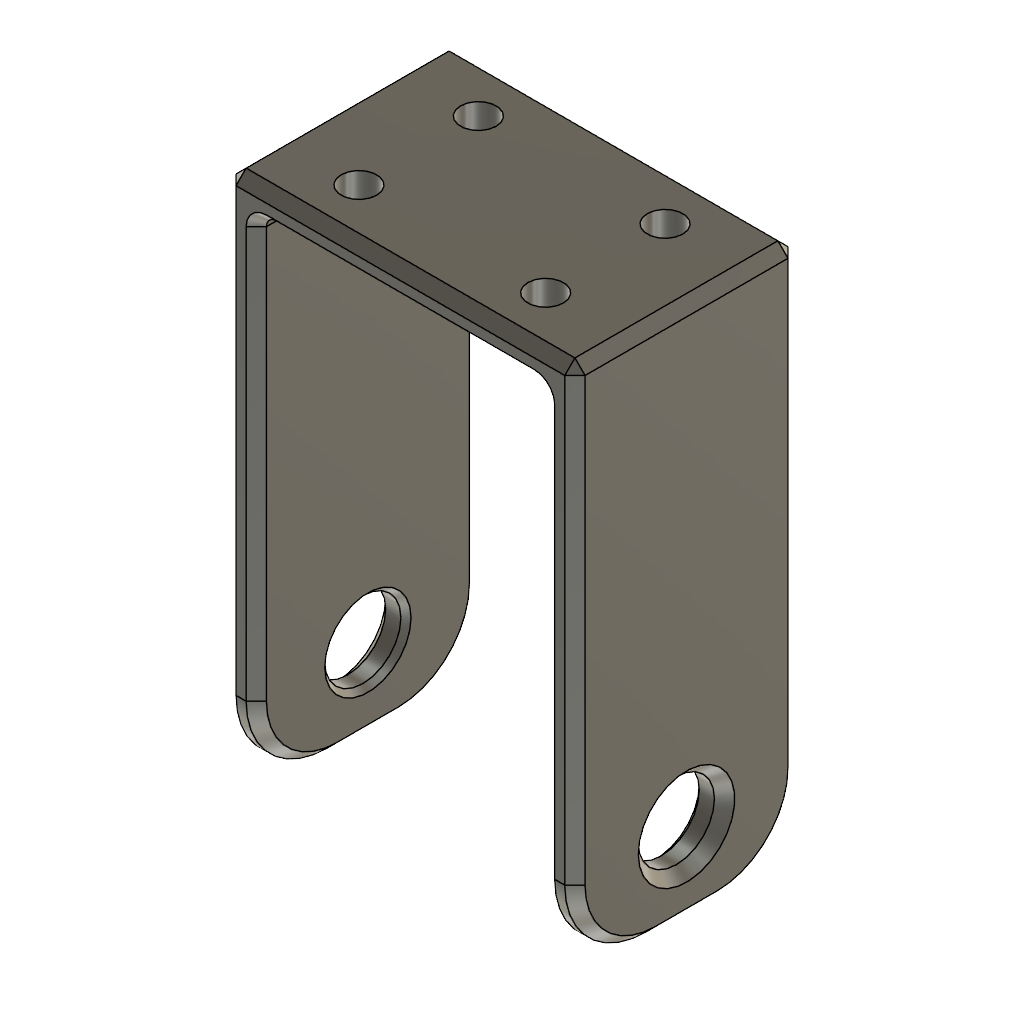
ZoMa_Bracket_omni_wheel_v001 (Autodesk Fusion 360 design; units mm, degrees)
part number: 2026-08-14-10-01-13-584
part number: 2026-08-14-10-48-38-713
part number: 2026-08-14-10-49-42-886
part number: 2026-08-14-10-49-47-612
part number: 2026-08-14-10-49-51-894
part number: 2026-08-14-11-24-35-038
part number: 2026-08-18-17-26-55-880
part number: 2026-08-18-17-40-12-881
part number: 2026-08-19-15-49-04-728
part number: 2026-08-21-16-16-46-057
part number: 2026-08-21-16-33-57-541
part number: 2026-08-21-17-08-07-984
part number: 2026-08-21-22-58-38-714
part number: 2026-08-22-15-22-42-177
part number: 2026-08-22-15-58-47-790
part number: 2026-08-23-22-18-51-194
part number: 2026-08-25-18-38-39-013
part number: 2026-08-25-18-59-01-897
Autodesk Fusion 360 part; units mm, degrees
note: some values were not read from the file. Set by a fixed rule: which sketch regions a step uses.
(part 1 of 2)
sketch "top_bracket" plane through (0, 0, 0) normal (0, 0, 1) x (1, 0, 0)
  line L0 (17.2, -11) -> (-17.2, -11)
  line L1 (-17.2, -11) -> (-17.2, 11)
  line L2 (-17.2, 11) -> (17.2, 11)
  line L3 (17.2, 11) -> (17.2, -11)
  line L4 (17.2, -11) -> (-17.2, 11) construction
  line L5 (-17.2, -11) -> (17.2, 11) construction
  line L6 (-9.2, 5.8837) -> (9.2, 5.8837) construction
  line L7 (9.2, 5.8837) -> (9.2, -5.8837) construction
  line L8 (9.2, -5.8837) -> (-9.2, -5.8837) construction
  line L9 (-9.2, -5.8837) -> (-9.2, 5.8837) construction
  circle A0 centre (-9.2, 5.8837) radius 1.75
  circle A1 centre (9.2, 5.8837) radius 1.75
  circle A2 centre (9.2, -5.8837) radius 1.75
  circle A3 centre (-9.2, -5.8837) radius 1.75
  dimension "d6" = 34.4
  dimension "d8" = 22
  dimension "d10" = 8
  dimension "d11" = 8
  dimension "d12" = 3.5
  dimension "d13" = 3.5
  dimension "d14" = 3.5
  dimension "d15" = 3.5
  dimension "d56" = 18.4
  dimension "d57" = 11.7674
  constraint horizontal L0
  constraint perpendicular L0 L1
  constraint parallel L0 L2
  constraint parallel L1 L3
  constraint coincident L4 origin
  constraint coincident L5 origin
  constraint horizontal L6
  constraint vertical L7
  constraint horizontal L8
  constraint vertical L9
  constraint coincident L4 L7.end
  constraint coincident L4 L6.start
  constraint coincident L6.start L9.end
  constraint coincident L6.end L7.start
  constraint coincident L7.end L8.start
  constraint coincident L8.end L9.start
  measures "d6" distance of L1.end L2.end
  measures "d8" distance of L0.end L1.end
  measures "d10" distance of L1 L9
  measures "d11" distance of L3 L7
  measures "d12" diameter of A0
  measures "d13" diameter of A1
  measures "d14" diameter of A2
  measures "d15" diameter of A3
  measures "d56" distance of L6.start L6.end
  measures "d57" distance of L6.end L7.end
sketch "side_bracket_1" plane through (0, 0, 0) normal (1, 0, 0) x (0, 1, 0)
  line L0 (11, -24.75) -> (-11, -24.75)
  line L1 (-11, -24.75) -> (-11, 24.75)
  line L2 (-11, 24.75) -> (11, 24.75)
  line L3 (11, 24.75) -> (11, -24.75)
  line L4 (11, -24.75) -> (-11, 24.75) construction
  line L5 (-11, -24.75) -> (11, 24.75) construction
  line L6 (0, 24.75) -> (0, -24.75) construction
  circle A0 centre (0, -16.75) radius 3.75
  dimension "d16" = 22
  dimension "d17" = 49.5
  dimension "d20" = 7.5
  dimension "d21" = 41.5
  constraint horizontal L0
  constraint perpendicular L0 L1
  constraint parallel L0 L2
  constraint parallel L1 L3
  constraint coincident L4 origin
  constraint coincident L5 origin
  constraint midpoint L2 L6.start
  constraint midpoint L0 L6.end
  constraint coincident L6 A0.centre
  measures "d16" distance of L1.end L2.end
  measures "d17" distance of L0.end L1.end
  measures "d20" diameter of A0
  measures "d21" distance of L2 A0.centre
extrude "Extrude1" add sketch "side_bracket_1" along normal blind 3 makes body 1
sketch "flange" plane through (3, 0, 0) normal (1, 0, 0) x (0, 1, 0)
  circle A0 centre (0, -16.75) radius 3.75
  line L0 (11, 24.75) -> (-11, 24.75)
  line L1 (-11, 24.75) -> (-11, -24.75)
  line L2 (-11, -24.75) -> (11, -24.75)
  line L3 (11, -24.75) -> (11, 24.75)
  circle A1 centre (0, -16.75) radius 4.25
  dimension "d24" = 8.5
  constraint concentric A0 A1
  measures "d24" diameter of A1
extrude "Extrude2" cut sketch "flange" against normal blind 0.5 contours A1 bodies 1
copy_body "CopyPasteBodies1" bodies 1 makes body 2
move_body "Move1" bodies 2 to x (1, 0, 0) y (0, 1, 0) z (0, 0, 1) at (-16.4295, -31.9665, 2.9129)
fillet "Fillet1" radius 8 4 edges at (1.5, -11, -24.75) (1.5, 11, -24.75) (-14.9295, -20.9665, -21.8371) (-14.9295, -42.9665, -21.8371) on bodies 1 2
move_body "Move2" bodies 1 to x (1, 0, 0) y (0, 1, 0) z (0, 0, 1) at (8.0272, -22.7991, 0)
extrude "Extrude3" add sketch "top_bracket" along normal blind 3 separate body makes body 3
copy_body "CutPasteBodies1" bodies 1 2 3 removing the originals makes body 4 makes body 5 makes body 6 in component "bracket_omni_wheel"
copy_body "Body->Comp1" bodies 4 removing the originals makes body 7 in component "side_bracket_1"
copy_body "Body->Comp2" bodies 5 removing the originals makes body 8 in component "side_bracket_2"
copy_body "Body->Comp3" bodies 6 removing the originals makes body 9 in component "top_bracket"
combine "Combine1" operation add target body 7 tool bodies 9 8 body 9 seen with x (1, 0, 0) y (0, 1, 0) z (0, 0, 1) at (-6.1728, -22.7991, 24.75) body 8 seen with x (-1, 0, 0) y (0, -1, 0) z (0, 0, 1) at (-36.8023, -54.7656, -2.9129) in component "side_bracket_1"
fillet "Fillet1'" radius 1 2 edges at (-20.3728, -22.7991, 24.75) (8.0272, -22.7991, 24.75) on bodies 7 in component "side_bracket_1"
chamfer "Chamfer1" distance 1 angle 45 30 edges at (11.0272, -22.7991, 27.75) (-6.1728, -11.7991, 27.75) (-6.1728, -33.7991, 27.75) (-23.3728, -22.7991, 27.75) (-23.3728, -11.7991, 5.5) (-23.3728, -33.7991, 5.5) (-23.3728, -31.456, -22.4069) (-23.3728, -22.7991, -24.75) (-23.3728, -14.1423, -22.4069) (11.0272, -33.7991, 5.5) (11.0272, -11.7991, 5.5) (11.0272, -14.1423, -22.4069) (11.0272, -22.7991, -24.75) (11.0272, -31.456, -22.4069) (-6.1728, -11.7991, 24.75) (7.7343, -11.7991, 24.4571) (8.0272, -11.7991, 3.5) (8.0272, -14.1423, -22.4069) (8.0272, -22.7991, -24.75) (8.0272, -31.456, -22.4069) (8.0272, -33.7991, 3.5) (7.7343, -33.7991, 24.4571) (-6.1728, -33.7991, 24.75) (-20.0799, -33.7991, 24.4571) (-20.3728, -33.7991, 3.5) (-20.3728, -31.456, -22.4069) (-20.3728, -22.7991, -24.75) (-20.3728, -14.1423, -22.4069) (-20.3728, -11.7991, 3.5) (-20.0799, -11.7991, 24.4571) on bodies 7 in component "side_bracket_1"
sketch "chassis_bottom_deck" plane through (0, 0, 0) normal (0, 0, 1) x (1, 0, 0) in component "chassis_bottom_deck"
  line L0 (150, -150) -> (-150, -150)
  line L1 (-150, -150) -> (-150, 150)
  line L2 (-150, 150) -> (150, 150)
  line L3 (150, 150) -> (150, -150)
  line L4 (150, -150) -> (-150, 150) construction
  line L5 (-150, -150) -> (150, 150) construction
  line L6 (-150, -30) -> (-115, -30)
  line L7 (-115, -30) -> (-115, -110)
  line L8 (-115, -110) -> (-150, -110)
  line L9 (-150, -110) -> (-150, -30)
  line L10 (-115, -70) -> (150, -70) construction
  line L11 (-73, -85) -> (-97, -85) construction
  line L12 (-97, -85) -> (-97, -55) construction
  line L13 (-97, -55) -> (-73, -55) construction
  line L14 (-73, -55) -> (-73, -85) construction
  line L15 (-73, -85) -> (-97, -55) construction
  line L16 (-97, -85) -> (-73, -55) construction
  line L17 (-58, -100) -> (-48, -100)
  line L18 (-48, -100) -> (-48, -110)
  line L19 (-48, -110) -> (-58, -110)
  line L20 (-58, -110) -> (-58, -100)
  line L21 (0, 150) -> (0, -150) construction
  line L22 (-120, 120) -> (-94.1, 120) construction
  line L23 (-94.1, 120) -> (-94.1, 72) construction
  line L24 (-94.1, 72) -> (-120, 72) construction
  line L25 (-120, 72) -> (-120, 120) construction
  line L26 (-107.05, 120) -> (-107.05, 72) construction
  line L27 (-94.1, 96) -> (-120, 96) construction
  line L28 (-97.85, 90.1163) -> (-116.25, 90.1163) construction
  line L29 (-116.25, 90.1163) -> (-116.25, 101.8837) construction
  line L30 (-116.25, 101.8837) -> (-97.85, 101.8837) construction
  line L31 (-97.85, 101.8837) -> (-97.85, 90.1163) construction
  line L32 (-97.85, 90.1163) -> (-116.25, 101.8837) construction
  line L33 (-116.25, 90.1163) -> (-97.85, 101.8837) construction
  circle A0 centre (-116.25, 101.8837) radius 1.5
  circle A1 centre (-97.85, 101.8837) radius 1.5
  circle A2 centre (-97.85, 90.1163) radius 1.5
  circle A3 centre (-116.25, 90.1163) radius 1.5
  circle A4 centre (-97, -55) radius 1.5
  circle A5 centre (-73, -55) radius 1.5
  circle A6 centre (-73, -85) radius 1.5
  circle A7 centre (-97, -85) radius 1.5
  circle A8 centre (73, -55) radius 1.5
  circle A9 centre (97, -55) radius 1.5
  line L34 (150, -110) -> (150, -30)
  line L35 (150, -30) -> (115, -30)
  line L36 (115, -30) -> (115, -110)
  line L37 (115, -110) -> (150, -110)
  circle A10 centre (73, -85) radius 1.5
  circle A11 centre (97, -85) radius 1.5
  circle A12 centre (97.85, 101.8837) radius 1.5
  circle A13 centre (97.85, 90.1163) radius 1.5
  circle A14 centre (116.25, 90.1163) radius 1.5
  circle A15 centre (116.25, 101.8837) radius 1.5
  line L38 (48, -30) -> (58, -30)
  line L39 (58, -30) -> (58, -40)
  line L40 (58, -40) -> (48, -40)
  line L41 (48, -40) -> (48, -30)
  point P0 (-85, -70)
  point P1 (-107.05, 96)
  dimension "d42" = 300
  dimension "d43" = 300
  dimension "d44" = 35
  dimension "d45" = 80
  dimension "d46" = 40
  dimension "d47" = 24
  dimension "d48" = 30
  dimension "d49" = 53
  dimension "d50" = 10
  dimension "d51" = 10
  dimension "d52" = 15
  dimension "d53" = 15
  dimension "d54" = 25.9
  dimension "d55" = 48
  dimension "d58" = 18.4
  dimension "d59" = 11.7674
  dimension "d60" = 30
  dimension "d61" = 30
  dimension "d62" = 3
  dimension "d63" = 3
  dimension "d64" = 3
  dimension "d65" = 3
  dimension "d66" = 3
  dimension "d67" = 3
  dimension "d68" = 3
  dimension "d69" = 3
  dimension "d70" = 10
  dimension "d71" = 10
  dimension "d72" = 15
  dimension "d73" = 15
  constraint horizontal L0
  constraint perpendicular L0 L1
  constraint parallel L0 L2
  constraint parallel L1 L3
  constraint coincident L4 origin
  constraint coincident L5 origin
  constraint horizontal L6
  constraint vertical L7
  constraint horizontal L8
  constraint vertical L9
  constraint coincident L1 L6.start
  constraint midpoint L7 L10.start
  constraint coincident L3 L10.end
  constraint perpendicular L3 L10
  constraint horizontal L11
  constraint perpendicular L11 L12
  constraint parallel L11 L13
  constraint parallel L12 L14
  constraint coincident L15 P0
  constraint coincident L16 P0
  constraint coincident L10 P0
  constraint horizontal L17
  constraint vertical L18
  constraint horizontal L19
  constraint vertical L20
  constraint midpoint L2 L21.start
  constraint midpoint L0 L21.end
  constraint horizontal L22
  constraint vertical L23
  constraint horizontal L24
  constraint vertical L25
  constraint midpoint L22 L26.start
  constraint midpoint L24 L26.end
  constraint midpoint L23 L27.start
  constraint midpoint L25 L27.end
  constraint horizontal L28
  constraint perpendicular L28 L29
  constraint parallel L28 L30
  constraint parallel L29 L31
  constraint coincident L32 P1
  constraint coincident L33 P1
  constraint midpoint L26 P1
  constraint coincident L29.end L30.start
  constraint coincident L30.end L31.start
  constraint coincident L28.start L31.end
  constraint coincident L28.end L29.start
  constraint coincident L12.end L13.start
  constraint coincident L13.end L14.start
  constraint coincident L11.start L14.end
  constraint coincident L11.end L12.start
  constraint symmetric L6.start L21 L34.end
  constraint symmetric L6.end L21 L35.end
  constraint symmetric L7.end L21 L36.end
  constraint symmetric L8.end L21 L34.start
  constraint symmetric L21 A0 A15
  constraint symmetric L21 A1 A12
  constraint symmetric L21 A2 A13
  constraint symmetric L21 A3 A14
  constraint symmetric L21 A4 A9
  constraint symmetric L21 A5 A8
  constraint symmetric L21 A6 A10
  constraint symmetric L21 A7 A11
  constraint horizontal L38
  constraint vertical L39
  constraint horizontal L40
  constraint vertical L41
  measures "d42" distance of L0.end L1.end
  measures "d43" distance of L1.end L2.end
  measures "d44" distance of L6.start L6.end
  measures "d45" distance of L6.start L8.end
  measures "d46" distance of L0 L8
  measures "d47" distance of L12.end L13.end
  measures "d48" distance of L11.end L12.end
  measures "d49" distance of L9 L12
  measures "d50" distance of L17.start L17.end
  measures "d51" distance of L17.start L19.end
  measures "d52" distance of L14 L20
  measures "d53" distance of L11 L17
  measures "d54" distance of L22.start L22.end
  measures "d55" distance of L22.start L24.end
  measures "d58" distance of L29.end L30.end
  measures "d59" distance of L28.end L29.end
  measures "d60" distance of L1 L25
  measures "d61" distance of L2 L22
  measures "d62" diameter of A0
  measures "d63" diameter of A1
  measures "d64" diameter of A2
  measures "d65" diameter of A3
  measures "d66" diameter of A4
  measures "d67" diameter of A5
  measures "d68" diameter of A6
  measures "d69" diameter of A7
  measures "d70" distance of L38.start L38.end
  measures "d71" distance of L38.start L40.end
  measures "d72" distance of A8.centre L40
  measures "d73" distance of A8.centre L39
extrude "Extrude1'" add sketch "chassis_bottom_deck" along normal blind 3 separate body contours L0 L1 L2 L3 L6 L7 L8 L35 L36 L37 makes body 10 in component "chassis_bottom_deck"
sketch "Sketch1" plane through (0, 0, 0) normal (0, 0, 1) x (1, 0, 0) in component "chassis_top_deck"
  line L0 (150, 150) -> (-150, 150)
  line L1 (-150, 150) -> (-150, -150)
  line L2 (-150, -150) -> (150, -150)
  line L3 (150, -150) -> (150, 150)
  line L4 (150, 150) -> (-150, -150) construction
  line L5 (-150, 150) -> (150, -150) construction
  line L6 (19.6, -17.5) -> (-19.6, -17.5)
  line L7 (-19.6, -17.5) -> (-19.6, 17.5)
  line L8 (-19.6, 17.5) -> (19.6, 17.5)
  line L9 (19.6, 17.5) -> (19.6, -17.5)
  line L10 (19.6, -17.5) -> (-19.6, 17.5) construction
  line L11 (-19.6, -17.5) -> (19.6, 17.5) construction
  line L12 (-122.4527, -20.5512) -> (-73.4527, -20.5512) construction
  line L13 (-73.4527, -20.5512) -> (-73.4527, -78.5512) construction
  line L14 (-73.4527, -78.5512) -> (-122.4527, -78.5512) construction
  line L15 (-122.4527, -78.5512) -> (-122.4527, -20.5512) construction
  circle A0 centre (-122.4527, -20.5512) radius 1.25
  circle A1 centre (-73.4527, -20.5512) radius 1.25
  circle A2 centre (-122.4527, -78.5512) radius 1.25
  circle A3 centre (-73.4527, -78.5512) radius 1.25
  dimension "d78" = 300
  dimension "d79" = 300
  dimension "d80" = 39.2
  dimension "d81" = 35
  dimension "d82" = 58
  dimension "d83" = 49
  dimension "d84" = 2.5
  dimension "d85" = 2.5
  dimension "d86" = 2.5
  dimension "d87" = 2.5
  constraint horizontal L0
  constraint perpendicular L0 L1
  constraint parallel L0 L2
  constraint parallel L1 L3
  constraint coincident L4 origin
  constraint coincident L5 origin
  constraint horizontal L6
  constraint perpendicular L6 L7
  constraint parallel L6 L8
  constraint parallel L7 L9
  constraint coincident L10 origin
  constraint coincident L11 origin
  constraint horizontal L12
  constraint vertical L13
  constraint horizontal L14
  constraint vertical L15
  constraint coincident L12.start L15.end
  constraint coincident L12.end L13.start
  constraint coincident L14.end L15.start
  constraint coincident L13.end L14.start
  measures "d78" distance of L1.end L2.end
  measures "d79" distance of L0.end L1.end
  measures "d80" distance of L7.end L8.end
  measures "d81" distance of L6.end L7.end
  measures "d82" distance of L12.start L14.end
  measures "d83" distance of L12.start L12.end
  measures "d84" diameter of A0
  measures "d85" diameter of A1
  measures "d86" diameter of A2
  measures "d87" diameter of A3
sketch "Sketch1 (2)" plane through (0, 0, 0) normal (0, 0, 1) x (1, 0, 0) in component "deck_vertical_spacer"
  circle A0 centre (0, 0) radius 5
  dimension "d88" = 10
  constraint coincident A0.centre origin
  measures "d88" diameter of A0
extrude "Extrude1''" add sketch "Sketch1 (2)" along normal blind 60 separate body makes body 11 in component "deck_vertical_spacer"
sketch "Sketch4" plane through (0, 0, 60) normal (0, 0, 1) x (-1, 0, 0) in component "deck_vertical_spacer"
  circle A0 centre (0, 0) radius 5
  circle A1 centre (0, 0) radius 2
  dimension "d97" = 4
  constraint coincident A0.centre A1.centre
  measures "d97" diameter of A1
extrude "Extrude3'" cut sketch "Sketch4" against normal blind 15 contours A1 bodies 11 in component "deck_vertical_spacer"
chamfer "Chamfer2" distance 0.5 angle 45 6 edges at (-20.3728, -19.3029, -15.3939) (10.5272, -26.2953, -18.1061) (8.0272, -26.2953, -15.3939) (11.0272, -26.7615, -15.2131) (-22.8728, -19.3029, -18.1061) (-23.3728, -18.8367, -15.2131) on bodies 7 in component "side_bracket_1"
chamfer "Chamfer3" distance 0.5 angle 45 4 edges at (-17.0044, -28.05, 24.75) (1.3956, -28.05, 24.75) (1.3956, -16.2826, 24.75) (-17.0044, -16.2826, 24.75) on bodies 7 in component "side_bracket_1"
sketch "Sketch1 (3)" plane through (0, 0, 0) normal (0, 0, 1) x (1, 0, 0) in component "component_spacer"
  circle A0 centre (0, 0) radius 3.05
  dimension "d109" = 6.1
  constraint coincident A0.centre origin
  measures "d109" diameter of A0
extrude "Extrude1'''" add sketch "Sketch1 (3)" along normal blind 12 separate body makes body 12 in component "component_spacer"
sketch "Sketch2" plane through (0, 0, 12) normal (0, 0, 1) x (-1, 0, 0) in component "component_spacer"
  circle A0 centre (0, 0) radius 3.05
  circle A1 centre (0, 0) radius 1.15
  dimension "d112" = 2.3
  constraint coincident A0.centre A1.centre
  measures "d112" diameter of A1
extrude "Extrude2'" cut sketch "Sketch2" against normal blind 12 contours A1 bodies 12 in component "component_spacer"
chamfer "Chamfer1'" distance 0.4 angle 45 1 edges at (1.0722, 0.4159, 0) on bodies 12 in component "component_spacer"
sketch "Sketch1 (4)" plane through (0, 0, 0) normal (0, 0, 1) x (1, 0, 0) in component "profile_square"
  line L0 (18, -18) -> (-18, -18)
  line L1 (-18, -18) -> (-18, 18)
  line L2 (-18, 18) -> (18, 18)
  line L3 (18, 18) -> (18, -18)
  line L4 (18, -18) -> (-18, 18) construction
  line L5 (-18, -18) -> (18, 18) construction
  line L6 (14, -14) -> (-14, -14)
  line L7 (-14, -14) -> (-14, 14)
  line L8 (-14, 14) -> (14, 14)
  line L9 (14, 14) -> (14, -14)
  line L10 (14, -14) -> (-14, 14) construction
  line L11 (-14, -14) -> (14, 14) construction
  dimension "d119" = 36
  dimension "d120" = 36
  dimension "d121" = 28
  dimension "d122" = 28
  constraint horizontal L0
  constraint perpendicular L0 L1
  constraint parallel L0 L2
  constraint parallel L1 L3
  constraint coincident L4 origin
  constraint coincident L5 origin
  constraint horizontal L6
  constraint perpendicular L6 L7
  constraint parallel L6 L8
  constraint parallel L7 L9
  constraint coincident L10 origin
  constraint coincident L11 origin
  measures "d119" distance of L1.end L2.end
  measures "d120" distance of L0.end L1.end
  measures "d121" distance of L7.end L8.end
  measures "d122" distance of L6.end L7.end
sketch "Sketch1 (5)" plane through (0, 0, 0) normal (0, 0, 1) x (1, 0, 0) in component "profile_rectangle"
  line L0 (6, -10.4) -> (-6, -10.4)
  line L1 (-6, -10.4) -> (-6, 10.4)
  line L2 (-6, 10.4) -> (6, 10.4)
  line L3 (6, 10.4) -> (6, -10.4)
  line L4 (6, -10.4) -> (-6, 10.4) construction
  line L5 (-6, -10.4) -> (6, 10.4) construction
  line L6 (-9, 18.4) -> (9, 18.4)
  line L7 (9, 18.4) -> (9, -13.4)
  line L8 (9, -13.4) -> (-9, -13.4)
  line L9 (-9, -13.4) -> (-9, 18.4)
  dimension "d276" = 12
  dimension "d277" = 20.8
  dimension "d278" = 3
  dimension "d279" = 3
  dimension "d280" = 3
  dimension "d281" = 8
  constraint horizontal L0
  constraint perpendicular L0 L1
  constraint parallel L0 L2
  constraint parallel L1 L3
  constraint coincident L4 origin
  constraint coincident L5 origin
  constraint horizontal L6
  constraint vertical L7
  constraint horizontal L8
  constraint vertical L9
  measures "d276" distance of L1.end L2.end
  measures "d277" distance of L0.end L1.end
  measures "d278" distance of L3 L7
  measures "d279" distance of L1 L9
  measures "d280" distance of L0 L8
  measures "d281" distance of L2 L6
extrude "Extrude1''''" add sketch "Sketch1 (5)" against normal blind 1 separate body makes body 13 in component "profile_rectangle"
sketch "Sketch2 (2)" plane through (0, 0, 0) normal (0, 0, 1) x (-1, 0, 0) in component "profile_rectangle"
  line L0 (6, -10.4) -> (-6, -10.4)
  line L1 (-6, -10.4) -> (-6, 10.4)
  line L2 (-6, 10.4) -> (6, 10.4)
  line L3 (6, 10.4) -> (6, -10.4)
  line L4 (9, 13.4) -> (-9, 13.4)
  line L5 (-9, 13.4) -> (-9, -18.4)
  line L6 (-9, -18.4) -> (9, -18.4)
  line L7 (9, -18.4) -> (9, 13.4)
  line L8 (6, -10.4) -> (-6, -10.4)
  line L9 (-6, -10.4) -> (-6, 10.4)
  line L10 (-6, 10.4) -> (6, 10.4)
  line L11 (6, 10.4) -> (6, -10.4)
  constraint horizontal L8
  constraint vertical L9
  constraint horizontal L10
  constraint vertical L11
  constraint coincident L1.end L2.start
  constraint coincident L0.start L3.end
sketch "Sketch1 (6)" plane through (0, 0, 0) normal (0, 0, 1) x (1, 0, 0) in component "profile_switch"
  line L0 (6, -10.15) -> (-6, -10.15)
  line L1 (-6, -10.15) -> (-6, 10.15)
  line L2 (-6, 10.15) -> (6, 10.15)
  line L3 (6, 10.15) -> (6, -10.15)
  line L4 (6, -10.15) -> (-6, 10.15) construction
  line L5 (-6, -10.15) -> (6, 10.15) construction
  line L6 (-9, 13.15) -> (9, 13.15)
  line L7 (9, 13.15) -> (9, -13.15)
  line L8 (9, -13.15) -> (-9, -13.15)
  line L9 (-9, -13.15) -> (-9, 13.15)
  dimension "d293" = 12
  dimension "d294" = 20.3
  dimension "d295" = 3
  dimension "d296" = 3
  dimension "d297" = 3
  dimension "d298" = 3
  constraint horizontal L0
  constraint perpendicular L0 L1
  constraint parallel L0 L2
  constraint parallel L1 L3
  constraint coincident L4 origin
  constraint coincident L5 origin
  constraint horizontal L6
  constraint vertical L7
  constraint horizontal L8
  constraint vertical L9
  measures "d293" distance of L1.end L2.end
  measures "d294" distance of L0.end L1.end
  measures "d295" distance of L2 L6
  measures "d296" distance of L0 L8
  measures "d297" distance of L1 L9
  measures "d298" distance of L3 L7
extrude "Extrude1'''''" add sketch "Sketch1 (6)" along normal blind 1 separate body makes body 14 in component "profile_switch"
sketch "Sketch2 (3)" plane through (0, 0, 1) normal (0, 0, 1) x (-1, 0, 0) in component "profile_switch"
  line L0 (6, -10.15) -> (-6, -10.15)
  line L1 (-6, -10.15) -> (-6, 10.15)
  line L2 (-6, 10.15) -> (6, 10.15)
  line L3 (6, 10.15) -> (6, -10.15)
  line L4 (9, 13.15) -> (-9, 13.15)
  line L5 (-9, 13.15) -> (-9, -13.15)
  line L6 (-9, -13.15) -> (9, -13.15)
  line L7 (9, -13.15) -> (9, 13.15)
  line L8 (6, -10.15) -> (-6, -10.15)
  line L9 (-6, -10.15) -> (-6, 10.15)
  line L10 (-6, 10.15) -> (6, 10.15)
  line L11 (6, 10.15) -> (6, -10.15)
  constraint horizontal L8
  constraint vertical L9
  constraint horizontal L10
  constraint vertical L11
  constraint coincident L1.end L2.start
  constraint coincident L0.start L3.end
extrude "Extrude2''" add sketch "Sketch2 (3)" against normal blind 4 thin wall 0.5 inside contours L0 L1 L2 L3 L8 L9 L10 L11 bodies 14 in component "profile_switch"
fillet "Fillet2" radius 2 4 edges at (-9, -13.15, 0.5) (-9, 13.15, 0.5) (9, -13.15, 0.5) (9, 13.15, 0.5) on bodies 14 in component "profile_switch"
sketch "Sketch3" plane through (0, 0, 1) normal (0, 0, 1) x (-1, 0, 0) in component "profile_switch"
  line L0 (-5.5, -9.65) -> (-5.5, 9.65)
  line L1 (-5.5, 9.65) -> (5.5, 9.65)
  line L2 (5.5, 9.65) -> (5.5, -9.65)
  line L3 (5.5, -9.65) -> (-5.5, -9.65)
  arc A0 (-9, -11.15) -> (-7, -13.15) centre (-7, -11.15) ccw
  line L4 (-7, -13.15) -> (7, -13.15)
  arc A1 (7, -13.15) -> (9, -11.15) centre (7, -11.15) ccw
  line L5 (9, -11.15) -> (9, 11.15)
  arc A2 (9, 11.15) -> (7, 13.15) centre (7, 11.15) ccw
  line L6 (7, 13.15) -> (-7, 13.15)
  arc A3 (-7, 13.15) -> (-9, 11.15) centre (-7, 11.15) ccw
  line L7 (-9, 11.15) -> (-9, -11.15)
  line L8 (5.5, -9.65) -> (-5.5, -9.65)
  line L9 (-5.5, -9.65) -> (-5.5, 9.65)
  line L10 (-5.5, 9.65) -> (5.5, 9.65)
  line L11 (5.5, 9.65) -> (5.5, -9.65)
  constraint horizontal L8
  constraint vertical L9
  constraint horizontal L10
  constraint vertical L11
  constraint coincident L0.end L1.start
  constraint coincident L2.end L3.start
extrude "Extrude3''" add sketch "Sketch3" against normal blind 1 contours L0 L1 L2 L3 L8 L9 L10 L11 bodies 14 in component "profile_switch"
fillet "Fillet4" radius 2 4 edges at (-9, 18.4, -0.5) (9, 18.4, -0.5) (-9, -13.4, -0.5) (9, -13.4, -0.5) on bodies 13 in component "profile_rectangle"
extrude "Extrude1''''''" [suppressed] in component "profile_square"
sketch "Sketch2 (4)" plane through (0, 0, 1) normal (0, 0, 1) x (-1, 0, 0) in component "profile_square"
  line L0 (14, -14) -> (-14, -14)
  line L1 (-14, -14) -> (-14, 14)
  line L2 (-14, 14) -> (14, 14)
  line L3 (14, 14) -> (14, -14)
  line L4 (-18, -18) -> (18, -18)
  line L5 (18, -18) -> (18, 18)
  line L6 (18, 18) -> (-18, 18)
  line L7 (-18, 18) -> (-18, -18)
  line L8 (-14.75, 14.75) -> (14.75, 14.75)
  line L9 (14.75, 14.75) -> (14.75, -14.75)
  line L10 (14.75, -14.75) -> (-14.75, -14.75)
  line L11 (-14.75, -14.75) -> (-14.75, 14.75)
  line L12 (-14.75, 14.75) -> (14.75, -14.75) construction
  line L13 (14.75, 14.75) -> (-14.75, -14.75) construction
  dimension "d125" = 29.5
  dimension "d126" = 29.5
  constraint horizontal L8
  constraint perpendicular L8 L9
  constraint parallel L8 L10
  constraint parallel L9 L11
  constraint coincident L12 origin
  constraint coincident L13 origin
  measures "d125" distance of L9.end L10.end
  measures "d126" distance of L8.end L9.end
extrude "Extrude2'''" [suppressed] in component "profile_square"
chamfer "Chamfer1''" [suppressed] in component "profile_square"
fillet "Fillet1''" [suppressed] in component "profile_square"
sketch "Sketch1 (7)" plane through (0, 0, 0) normal (0, 0, 1) x (1, 0, 0) in component "profile_rear_wheel"
  line L0 (44, 19.5) -> (-44, 19.5)
  line L1 (-44, 19.5) -> (-44, -19.5)
  line L2 (-44, -19.5) -> (44, -19.5)
  line L3 (44, -19.5) -> (44, 19.5)
  line L4 (44, 19.5) -> (-44, -19.5) construction
  line L5 (-44, 19.5) -> (44, -19.5) construction
  line L6 (-39, 28) -> (39, 28)
  line L7 (39, 28) -> (39, -14.5)
  line L8 (39, -14.5) -> (-39, -14.5)
  line L9 (-39, -14.5) -> (-39, 28)
  dimension "d134" = 88
  dimension "d135" = 39
  dimension "d136" = 5
  dimension "d137" = 5
  dimension "d138" = 5
  constraint horizontal L0
  constraint perpendicular L0 L1
  constraint parallel L0 L2
  constraint parallel L1 L3
  constraint coincident L4 origin
  constraint coincident L5 origin
  constraint horizontal L6
  constraint vertical L7
  constraint horizontal L8
  constraint vertical L9
  measures "d134" distance of L1.end L2.end
  measures "d135" distance of L0.end L1.end
  measures "d136" distance of L1 L9
  measures "d137" distance of L3 L7
  measures "d138" distance of L2 L8
extrude "Extrude1'''''''" [suppressed] in component "profile_rear_wheel"
sketch "Sketch2 (5)" plane through (0, 0, 1) normal (0, 0, 1) x (-1, 0, 0) in component "profile_rear_wheel"
  line L0 (39, 14.5) -> (39, -19.5)
  line L1 (39, -19.5) -> (44, -19.5)
  line L2 (44, -19.5) -> (44, 19.5)
  line L3 (44, 19.5) -> (-44, 19.5)
  line L4 (-44, 19.5) -> (-44, -19.5)
  line L5 (-44, -19.5) -> (-39, -19.5)
  line L6 (-39, -19.5) -> (-39, 14.5)
  line L7 (-39, 14.5) -> (39, 14.5)
  line L8 (40.5, -20) -> (-40.5, -20)
  line L9 (-40.5, -20) -> (-40.5, 16)
  line L10 (-40.5, 16) -> (40.5, 16)
  line L11 (40.5, 16) -> (40.5, -20)
  dimension "d141" = 3.5
  dimension "d142" = 3.5
  dimension "d143" = 3.5
  constraint horizontal L8
  constraint vertical L9
  constraint horizontal L10
  constraint vertical L11
  measures "d141" distance of L2 L11
  measures "d142" distance of L4 L9
  measures "d143" distance of L3 L10
extrude "Extrude2''''" [suppressed] in component "profile_rear_wheel"
fillet "Fillet1'''" [suppressed] in component "profile_rear_wheel"
chamfer "Chamfer1'''" [suppressed] in component "profile_rear_wheel"
sketch "Sketch1 (8)" plane through (0, 0, 0) normal (0, 0, 1) x (1, 0, 0) in component "profile_corners"
  circle A0 centre (0, 0) radius 33
  circle A1 centre (0, 0) radius 38
  line L0 (0, 38) -> (0, 0)
  line L1 (0, 0) -> (38, 0)
  dimension "d151" = 66
  dimension "d152" = 76
  constraint coincident A0.centre A1.centre
  constraint concentric A0 A1
  constraint coincident A1 L0.start
  constraint vertical L0
  constraint coincident A1 L1.end
  constraint perpendicular L0 L1
  measures "d151" diameter of A0
  measures "d152" diameter of A1
extrude "Extrude1''''''''" [suppressed] in component "profile_corners"
sketch "Sketch3 (2)" plane through (0, 0, 1) normal (0, 0, 1) x (-1, 0, 0) in component "profile_corners"
  arc A0 (-38, 0) -> (0, -38) centre (0, 0) ccw
  line L0 (0, -38) -> (0, -33)
  arc A1 (-33, 0) -> (0, -33) centre (0, 0) ccw
  line L1 (-33, 0) -> (-38, 0)
  circle A2 centre (0, 0) radius 36.5
  dimension "d156" = 73
  dimension "d164" = 1.5
  dimension "d165" = 3.5
  constraint concentric A0 A2
  measures "d156" diameter of A2
  measures "d164" distance of A0 A2
  measures "d165" distance of A1 A2
extrude "Extrude2'''''" [suppressed] in component "profile_corners"
fillet "Fillet1''''" [suppressed] in component "profile_corners"
chamfer "Chamfer1''''" [suppressed] in component "profile_corners"
chamfer "Chamfer2'" [suppressed] in component "profile_corners"
chamfer "Chamfer3'" [suppressed] in component "profile_corners"
thread "Thread3" [suppressed] in component "deck_vertical_spacer"
sketch "Sketch1 (9)" plane through (0, 0, 0) normal (0, 0, 1) x (1, 0, 0) in component "mast_base"
  line L0 (40, 40) -> (-40, 40)
  line L1 (-40, 40) -> (-40, -40)
  line L2 (-40, -40) -> (40, -40)
  line L3 (40, -40) -> (40, 40)
  line L4 (40, 40) -> (-40, -40) construction
  line L5 (-40, 40) -> (40, -40) construction
  line L6 (19, -19) -> (-19, -19)
  line L7 (-19, -19) -> (-19, 19)
  line L8 (-19, 19) -> (19, 19)
  line L9 (19, 19) -> (19, -19)
  line L10 (19, -19) -> (-19, 19) construction
  line L11 (-19, -19) -> (19, 19) construction
  dimension "d168" = 80
  dimension "d169" = 80
  dimension "d170" = 21
  dimension "d171" = 38
  constraint horizontal L0
  constraint perpendicular L0 L1
  constraint parallel L0 L2
  constraint parallel L1 L3
  constraint coincident L4 origin
  constraint coincident L5 origin
  constraint horizontal L6
  constraint perpendicular L6 L7
  constraint parallel L6 L8
  constraint parallel L7 L9
  constraint coincident L10 origin
  constraint coincident L11 origin
  constraint coincident L5 L6.start
  measures "d168" distance of L1.end L2.end
  measures "d169" distance of L0.end L1.end
  measures "d170" distance of L1 L7
  measures "d171" distance of L7.end L8.end
extrude "Extrude1'''''''''" [suppressed] in component "mast_base"
sketch "Sketch2 (6)" plane through (0, 0, 3) normal (0, 0, 1) x (-1, 0, 0) in component "mast_base"
  line L0 (19, -19) -> (-19, -19)
  line L1 (-19, -19) -> (-19, 19)
  line L2 (-19, 19) -> (19, 19)
  line L3 (19, 19) -> (19, -19)
  line L4 (-40, 40) -> (-40, -40)
  line L5 (-40, -40) -> (40, -40)
  line L6 (40, -40) -> (40, 40)
  line L7 (40, 40) -> (-40, 40)
  line L8 (-22, 22) -> (22, 22)
  line L9 (22, 22) -> (22, -22)
  line L10 (22, -22) -> (-22, -22)
  line L11 (-22, -22) -> (-22, 22)
  line L12 (-22, 22) -> (22, -22) construction
  line L13 (22, 22) -> (-22, -22) construction
  line L14 (-25, 25) -> (25, 25)
  line L15 (25, 25) -> (25, -25)
  line L16 (25, -25) -> (-25, -25)
  line L17 (-25, -25) -> (-25, 25)
  line L18 (-25, 25) -> (25, -25) construction
  line L19 (25, 25) -> (-25, -25) construction
  line L20 (-28, 28) -> (28, 28)
  line L21 (28, 28) -> (28, -28)
  line L22 (28, -28) -> (-28, -28)
  line L23 (-28, -28) -> (-28, 28)
  line L24 (-28, 28) -> (28, -28) construction
  line L25 (28, 28) -> (-28, -28) construction
  line L26 (19, -25) -> (19, -22)
  line L27 (22, -19) -> (25, -19)
  line L28 (22, 19) -> (25, 19)
  line L29 (19, 22) -> (19, 25)
  line L30 (-19, 22) -> (-19, 25)
  line L31 (-22, 19) -> (-25, 19)
  line L32 (-22, -19) -> (-25, -19)
  line L33 (-19, -22) -> (-19, -25)
  dimension "d174" = 3
  dimension "d175" = 3
  dimension "d176" = 3
  dimension "d177" = 38
  dimension "d178" = 38
  dimension "d179" = 38
  dimension "d180" = 38
  dimension "d181" = 38
  constraint horizontal L8
  constraint perpendicular L8 L9
  constraint parallel L8 L10
  constraint parallel L9 L11
  constraint coincident L12 origin
  constraint coincident L13 origin
  constraint horizontal L14
  constraint perpendicular L14 L15
  constraint parallel L14 L16
  constraint parallel L15 L17
  constraint coincident L18 origin
  constraint coincident L19 origin
  constraint horizontal L20
  constraint perpendicular L20 L21
  constraint parallel L20 L22
  constraint parallel L21 L23
  constraint coincident L24 origin
  constraint coincident L25 origin
  constraint coincident L16 L26.start
  constraint coincident L10 L26.end
  constraint perpendicular L10 L26
  constraint coincident L9 L27.start
  constraint coincident L15 L27.end
  constraint perpendicular L15 L27
  constraint coincident L9 L28.start
  constraint coincident L15 L28.end
  constraint perpendicular L15 L28
  constraint coincident L8 L29.start
  constraint coincident L14 L29.end
  constraint perpendicular L14 L29
  constraint coincident L8 L30.start
  constraint coincident L14 L30.end
  constraint perpendicular L14 L30
  constraint coincident L11 L31.start
  constraint coincident L17 L31.end
  constraint perpendicular L17 L31
  constraint coincident L11 L32.start
  constraint coincident L17 L32.end
  constraint perpendicular L17 L32
  constraint coincident L10 L33.start
  constraint coincident L16 L33.end
  constraint perpendicular L16 L33
  measures "d174" distance of L1 L11
  measures "d175" distance of L11 L17
  measures "d176" distance of L17 L23
  measures "d177" distance of L0.start L2.end
  measures "d178" distance of L27 L28
  measures "d179" distance of L26 L33
  measures "d180" distance of L31 L32
  measures "d181" distance of L29 L30
extrude "Extrude2''''''" [suppressed] in component "mast_base"
chamfer "Chamfer1'''''" [suppressed] in component "mast_base"
sketch "Sketch3 (3)" plane through (0, 0, 3) normal (0, 0, 1) x (-1, 0, 0) in component "mast_base"
  line L0 (38, -38) -> (38, 38)
  line L1 (38, 38) -> (-38, 38)
  line L2 (-38, 38) -> (-38, -38)
  line L3 (-38, -38) -> (38, -38)
  line L4 (-30, -30) -> (-30, 30)
  line L5 (-30, 30) -> (30, 30)
  line L6 (30, 30) -> (30, -30)
  line L7 (30, -30) -> (-30, -30)
  line L8 (38, 0) -> (30, 0)
  line L9 (0, -38) -> (0, -30)
  line L10 (-30, 0) -> (-38, 0)
  line L11 (0, 30) -> (0, 38)
  circle A0 centre (34, 0) radius 1.5
  circle A1 centre (0, -34) radius 1.5
  circle A2 centre (-34, 0) radius 1.5
  circle A3 centre (0, 34) radius 1.5
  dimension "d185" = 3
  dimension "d186" = 3
  dimension "d187" = 3
  dimension "d188" = 3
  constraint midpoint L0 L8.start
  constraint midpoint L6 L8.end
  constraint midpoint L3 L9.start
  constraint midpoint L7 L9.end
  constraint midpoint L4 L10.start
  constraint midpoint L2 L10.end
  constraint midpoint L5 L11.start
  constraint midpoint L1 L11.end
  constraint midpoint L8 A0.centre
  constraint midpoint L9 A1.centre
  constraint midpoint L10 A2.centre
  constraint midpoint L11 A3.centre
  measures "d185" diameter of A0
  measures "d186" diameter of A1
  measures "d187" diameter of A2
  measures "d188" diameter of A3
extrude "Extrude3'''" [suppressed] in component "mast_base"
fillet "Fillet1'''''" [suppressed] in component "mast_base"
chamfer "Chamfer2''" [suppressed] in component "mast_base"
sketch "Sketch2 (7)" plane through (0, 0, 1) normal (0, 0, 1) x (-1, 0, 0) in component "profile_corners"
  circle A0 centre (0, 0) radius 15
  line L0 (-0.1, -36.2999) -> (-0.1, -33.1998)
  arc A1 (-33.1998, -0.1) -> (-0.1, -33.1998) centre (0, 0) ccw
  line L1 (-33.1998, -0.1) -> (-36.2999, -0.1)
  arc A2 (-36.2999, -0.1) -> (-0.1, -36.2999) centre (0, 0) ccw
  constraint coincident A0.centre A1.centre
sketch "Sketch1 (10)" plane through (-14.2, 0, 0) normal (1, 0, 0) x (0, 1, 0) in component "bracket_omni_wheel"
  line L0 (-10, -1) -> (-10, -41.5)
  arc A0 (-10, -41.5) -> (-3, -48.5) centre (-3, -41.5) ccw
  line L1 (-3, -48.5) -> (3, -48.5)
  arc A1 (3, -48.5) -> (10, -41.5) centre (3, -41.5) ccw
  line L2 (10, -41.5) -> (10, -1)
  line L3 (10, -1) -> (-10, -1)
  circle A2 centre (0, -41.5) radius 4.25
  line L4 (-10, -7) -> (10, -7)
  line L5 (10, -7) -> (10, -10)
  line L6 (10, -10) -> (-10, -10)
  line L7 (-10, -10) -> (-10, -7)
  line L8 (-10, 0) -> (10, 0)
  dimension "d196" = 7
  constraint horizontal L4
  constraint vertical L5
  constraint horizontal L6
  constraint vertical L7
  constraint coincident L2 L5.end
  constraint coincident L0 L4.start
  measures "d196" distance of L4 L8
extrude "Extrude1''''''''''" [suppressed] in component "bracket_omni_wheel"
chamfer "Chamfer1''''''" [suppressed] in component "bracket_omni_wheel"
chamfer "Chamfer4" [suppressed] in component "side_bracket_1"
sketch "Sketch2 (8)" plane through (0, 0, 3) normal (0, 0, 1) x (-1, 0, 0) in component "bracket_omni_wheel"
  circle A0 centre (9.2, 5.8837) radius 2.25
  circle A1 centre (-9.2, 5.8837) radius 2.25
  line L0 (-16.2, 10) -> (-16.2, -10)
  line L1 (-16.2, -10) -> (16.2, -10)
  line L2 (16.2, -10) -> (16.2, 10)
  line L3 (16.2, 10) -> (-16.2, 10)
  circle A2 centre (-9.2, -5.8837) radius 2.25
  circle A3 centre (9.2, -5.8837) radius 2.25
  line L4 (9.2, -5.8837) -> (-9.2, -5.8837) construction
  line L5 (-9.2, -5.8837) -> (-9.2, 5.8837) construction
  line L6 (-9.2, 5.8837) -> (9.2, 5.8837) construction
  line L7 (9.2, 5.8837) -> (9.2, -5.8837) construction
  circle A4 centre (9.2, -5.8837) radius 1.75
  circle A5 centre (-9.2, -5.8837) radius 1.75
  circle A6 centre (-9.2, 5.8837) radius 1.75
  circle A7 centre (9.2, 5.8837) radius 1.75
  dimension "d202" = 3.5
  dimension "d203" = 3.5
  dimension "d204" = 3.5
  dimension "d205" = 3.5
  constraint coincident A3.centre L4.start
  constraint coincident A2.centre L4.end
  constraint coincident A1.centre L5.end
  constraint coincident A0.centre L6.end
  measures "d202" diameter of A4
  measures "d203" diameter of A5
  measures "d204" diameter of A6
  measures "d205" diameter of A7
extrude "Extrude2'''''''" [suppressed] in component "bracket_omni_wheel"
chamfer "Chamfer2'''" [suppressed] in component "bracket_omni_wheel"
sketch "Sketch1 (11)" plane through (0, 0, 0) normal (0, 0, 1) x (1, 0, 0) in component "deck_vertical_spacer_squared"
  line L0 (6, 6) -> (-6, 6)
  line L1 (-6, 6) -> (-6, -6)
  line L2 (-6, -6) -> (6, -6)
  line L3 (6, -6) -> (6, 6)
  line L4 (6, 6) -> (-6, -6) construction
  line L5 (-6, 6) -> (6, -6) construction
  dimension "d209" = 12
  dimension "d210" = 12
  constraint horizontal L0
  constraint perpendicular L0 L1
  constraint parallel L0 L2
  constraint parallel L1 L3
  constraint coincident L4 origin
  constraint coincident L5 origin
  measures "d209" distance of L1.end L2.end
  measures "d210" distance of L0.end L1.end
extrude "Extrude1'''''''''''" [suppressed] in component "deck_vertical_spacer_squared"
sketch "Sketch2 (9)" plane through (0, 0, 3) normal (0, 0, 1) x (-1, 0, 0) in component "deck_vertical_spacer_squared"
  line L0 (-6, 6) -> (-6, -6)
  line L1 (-6, -6) -> (6, -6)
  line L2 (6, -6) -> (6, 6)
  line L3 (6, 6) -> (-6, 6)
  line L4 (-6, 6) -> (6, 6)
  line L5 (6, 6) -> (6, -6)
  line L6 (6, -6) -> (-6, -6)
  line L7 (-6, -6) -> (-6, 6)
  line L8 (-6, 6) -> (6, -6) construction
  line L9 (6, 6) -> (-6, -6) construction
  constraint horizontal L4
  constraint perpendicular L4 L5
  constraint parallel L4 L6
  constraint parallel L5 L7
  constraint coincident L8 origin
  constraint coincident L9 origin
  constraint coincident L0.start L3.end
extrude "Extrude2''''''''" [suppressed] in component "deck_vertical_spacer_squared"
sketch "Sketch3 (4)" plane through (0, 0, 45) normal (0, 0, 1) x (-1, 0, 0) in component "deck_vertical_spacer_squared"
  line L0 (-4, -4) -> (-4, 4)
  line L1 (-4, 4) -> (4, 4)
  line L2 (4, 4) -> (4, -4)
  line L3 (4, -4) -> (-4, -4)
  line L4 (-6, -6) -> (6, -6)
  line L5 (6, -6) -> (6, 6)
  line L6 (6, 6) -> (-6, 6)
  line L7 (-6, 6) -> (-6, -6)
  line L8 (-6, 6) -> (6, 6)
  line L9 (6, 6) -> (6, -6)
  line L10 (6, -6) -> (-6, -6)
  line L11 (-6, -6) -> (-6, 6)
  line L12 (-6, 6) -> (6, -6) construction
  line L13 (6, 6) -> (-6, -6) construction
  constraint horizontal L8
  constraint perpendicular L8 L9
  constraint parallel L8 L10
  constraint parallel L9 L11
  constraint coincident L12 origin
  constraint coincident L13 origin
  constraint coincident L6.end L7.start
extrude "Extrude3''''" [suppressed] in component "deck_vertical_spacer_squared"
sketch "Sketch4 (2)" plane through (0, 0, 60) normal (0, 0, 1) x (-1, 0, 0) in component "deck_vertical_spacer_squared"
  line L0 (-6, -6) -> (6, -6)
  line L1 (6, -6) -> (6, 6)
  line L2 (6, 6) -> (-6, 6)
  line L3 (-6, 6) -> (-6, -6)
  circle A0 centre (0, 0) radius 1.45
  dimension "d218" = 2.9
  constraint coincident A0.centre origin
  measures "d218" diameter of A0
extrude "Extrude4" [suppressed] in component "deck_vertical_spacer_squared"
chamfer "Chamfer1'''''''" [suppressed] in component "deck_vertical_spacer_squared"
copy_body "CopyPasteBodies1'" [suppressed] in component "mast_base"
move_body "Move1'" [suppressed] in component "mast_base"
move_body "Move2'" [suppressed] in component "mast_base"
sketch "Sketch4 (3)" plane through (0, 0, 101.2478) normal (0, 0, 1) x (-1, 0, 0) in component "mast_base"
  line L0 (91.0824, -89.5035) -> (91.0824, -9.5035)
  line L1 (91.0824, -9.5035) -> (11.0824, -9.5035)
  line L2 (11.0824, -9.5035) -> (11.0824, -89.5035)
  line L3 (11.0824, -89.5035) -> (91.0824, -89.5035)
  line L4 (70.0824, -68.5035) -> (32.0824, -68.5035)
  line L5 (32.0824, -68.5035) -> (32.0824, -30.5035)
  line L6 (32.0824, -30.5035) -> (70.0824, -30.5035)
  line L7 (70.0824, -30.5035) -> (70.0824, -68.5035)
  circle A0 centre (51.0824, -15.5035) radius 1.5
  circle A1 centre (17.0824, -49.5035) radius 1.5
  circle A2 centre (85.0824, -49.5035) radius 1.5
  circle A3 centre (51.0824, -83.5035) radius 1.5
  line L8 (70.0824, -68.5035) -> (32.0824, -68.5035)
  line L9 (32.0824, -68.5035) -> (32.0824, -30.5035)
  line L10 (32.0824, -30.5035) -> (70.0824, -30.5035)
  line L11 (70.0824, -30.5035) -> (70.0824, -68.5035)
  constraint horizontal L8
  constraint vertical L9
  constraint horizontal L10
  constraint vertical L11
  constraint coincident L5.end L6.start
  constraint coincident L4.start L7.end
extrude "Extrude4'" [suppressed] in component "mast_base"
sketch "Sketch5" plane through (0, 0, 101.2478) normal (0, 0, 1) x (-1, 0, 0) in component "mast_base"
  line L0 (91.0824, -89.5035) -> (91.0824, -9.5035)
  line L1 (91.0824, -9.5035) -> (11.0824, -9.5035)
  line L2 (11.0824, -9.5035) -> (11.0824, -89.5035)
  line L3 (11.0824, -89.5035) -> (91.0824, -89.5035)
  circle A0 centre (51.0824, -15.5035) radius 1.5
  circle A1 centre (17.0824, -49.5035) radius 1.5
  circle A2 centre (85.0824, -49.5035) radius 1.5
  circle A3 centre (51.0824, -83.5035) radius 1.5
sketch "Sketch6" plane through (0, 0, 98.2478) normal (0, 0, -1) x (1, 0, 0) in component "mast_base"
  line L0 (-80.3752, -19.5035) -> (-21.7895, -19.5035)
  ellipse E0 centre (-22.4966, -20.9177) end of major axis (-21.2718, -19.693) minor radius 1 (-21.0824, -20.2106) -> (-21.7895, -19.5035) ccw
  line L1 (-21.0824, -20.2106) -> (-21.0824, -78.7964)
  ellipse E1 centre (-22.4966, -78.0893) end of major axis (-21.2718, -79.314) minor radius 1 (-21.7895, -79.5035) -> (-21.0824, -78.7964) ccw
  line L2 (-21.7895, -79.5035) -> (-80.3752, -79.5035)
  ellipse E2 centre (-79.6681, -78.0893) end of major axis (-80.8929, -79.314) minor radius 1 (-81.0824, -78.7964) -> (-80.3752, -79.5035) ccw
  line L3 (-81.0824, -78.7964) -> (-81.0824, -20.2106)
  ellipse E3 centre (-79.6681, -20.9177) end of major axis (-80.8929, -19.693) minor radius 1 (-80.3752, -19.5035) -> (-81.0824, -20.2106) ccw
  line L4 (-13.0824, -87.5035) -> (-13.0824, -11.5035)
  line L5 (-13.0824, -11.5035) -> (-89.0824, -11.5035)
  line L6 (-89.0824, -11.5035) -> (-89.0824, -87.5035)
  line L7 (-89.0824, -87.5035) -> (-13.0824, -87.5035)
  circle A0 centre (-51.0824, -15.5035) radius 1.5
  circle A1 centre (-17.0824, -49.5035) radius 1.5
  circle A2 centre (-85.0824, -49.5035) radius 1.5
  circle A3 centre (-51.0824, -83.5035) radius 1.5
sketch "Sketch7" plane through (0, 0, 98.2478) normal (0, 0, -1) x (1, 0, 0) in component "mast_base"
sketch "Sketch8" plane through (0, 0, 101.2478) normal (0, 0, 1) x (-1, 0, 0) in component "mast_base"
sketch "Sketch9" plane through (0, 0, 98.2478) normal (0, 0, -1) x (1, 0, 0) in component "mast_base"
copy_body "Body->Comp1'" [suppressed] in component "top_mast"
sketch "Sketch1 (12)" plane through (0, 0, 101.2478) normal (0, 0, 1) x (-1, 0, 0) in component "top_mast"
  line L0 (91.0824, -89.5035) -> (91.0824, -9.5035)
  line L1 (91.0824, -9.5035) -> (11.0824, -9.5035)
  line L2 (11.0824, -9.5035) -> (11.0824, -89.5035)
  line L3 (11.0824, -89.5035) -> (91.0824, -89.5035)
  circle A0 centre (51.0824, -15.5035) radius 1.5
  circle A1 centre (17.0824, -49.5035) radius 1.5
  circle A2 centre (85.0824, -49.5035) radius 1.5
  circle A3 centre (51.0824, -83.5035) radius 1.5
  line L4 (81.0824, -79.5035) -> (21.0824, -79.5035)
  line L5 (21.0824, -79.5035) -> (21.0824, -19.5035)
  line L6 (21.0824, -19.5035) -> (81.0824, -19.5035)
  line L7 (81.0824, -19.5035) -> (81.0824, -79.5035)
  dimension "d224" = 60
  dimension "d225" = 60
  dimension "d226" = 10
  dimension "d229" = 10
  dimension "d230" = 10
  dimension "d231" = 10
  constraint horizontal L4
  constraint vertical L5
  constraint horizontal L6
  constraint vertical L7
  measures "d224" distance of L4.start L6.end
  measures "d225" distance of L4.start L4.end
  measures "d226" distance of L3 L4
  measures "d229" distance of L1 L6
  measures "d230" distance of L2 L5
  measures "d231" distance of L0 L7
extrude "Extrude1''''''''''''" [suppressed] in component "top_mast"
chamfer "Chamfer1''''''''" [suppressed] in component "top_mast"
sketch "Sketch1 (13)" plane through (0, 0, 0) normal (0, 0, 1) x (1, 0, 0) in component "bumper_vertical"
  line L0 (10, 34.4) -> (-10, 34.4)
  line L1 (-10, 34.4) -> (-10, -34.4)
  line L2 (-10, -34.4) -> (10, -34.4)
  line L3 (10, -34.4) -> (10, 34.4)
  line L4 (10, 34.4) -> (-10, -34.4) construction
  line L5 (-10, 34.4) -> (10, -34.4) construction
  dimension "d251" = 68.8
  dimension "d252" = 20
  constraint horizontal L0
  constraint perpendicular L0 L1
  constraint parallel L0 L2
  constraint parallel L1 L3
  constraint coincident L4 origin
  constraint coincident L5 origin
  measures "d251" distance of L0.end L1.end
  measures "d252" distance of L0.start L0.end
extrude "Extrude1'''''''''''''" [suppressed] in component "bumper_vertical"
sketch "Sketch10" plane through (0, -34.4, 0) normal (0, -1, 0) x (1, 0, 0) in component "bumper_vertical"
  line L0 (-10, 0) -> (10, 0)
  line L1 (10, 0) -> (10, 1.5)
  line L2 (10, 1.5) -> (-10, 1.5)
  line L3 (-10, 1.5) -> (-10, 0)
sketch "Sketch11" plane through (0, 0, 1.5) normal (0, 0, 1) x (-1, 0, 0) in component "bumper_vertical"
  line L0 (-10, 34.4) -> (-10, -34.4)
  line L1 (-10, -34.4) -> (10, -34.4)
  line L2 (10, -34.4) -> (10, 34.4)
  line L3 (10, 34.4) -> (-10, 34.4)
  line L4 (10, 34.4) -> (-10.0697, 34.4)
  line L5 (-10.0697, 34.4) -> (-10.0697, 29)
  line L6 (-10.0697, 29) -> (10, 29)
  line L7 (10, 29) -> (10, 34.4)
  dimension "d263" = 5.4
  constraint horizontal L4
  constraint vertical L5
  constraint horizontal L6
  constraint vertical L7
  constraint coincident L2.end L3.start
  measures "d263" distance of L2.end L6.end
sketch "Sketch12" plane through (0, 0, 1.5) normal (0, 0, 1) x (-1, 0, 0) in component "bumper_vertical"
  line L0 (10, -34.4) -> (-10, -34.4)
  line L1 (-10, -34.4) -> (-10, -28.8)
  line L2 (-10, -28.8) -> (10, -28.8)
  line L3 (10, -28.8) -> (10, -34.4)
  point P0 (10, -34.4)
  dimension "d264" = 20
  dimension "d265" = 5.6
  constraint horizontal L0
  constraint vertical L1
  constraint horizontal L2
  constraint vertical L3
  constraint coincident P0 L0.start
  measures "d264" distance of P0 L0.end
  measures "d265" distance of P0 L2.end
extrude "Extrude4''" [suppressed] in component "bumper_vertical"